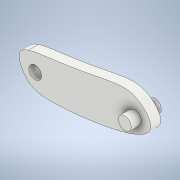
# Autodesk Inventor part: Component19
Saved by Autodesk Inventor 2022 (Build 260153000, 153)
## iProperties
Created: 2022-01-29
Part Number: Component19
Material: Generic
Document SubType Name: Modeling
Designer: Administrator
Density: 1 g/cm^3
Appearance: Default
Title: Component19
Author: Administrator
Autodesk Inventor part; units mm, degrees
ref_plane "YZ Plane" through (0, 0, 0) normal (1, 0, 0) x (0, 1, 0)
ref_plane "XZ Plane" through (0, 0, 0) normal (0, 1, 0) x (-1, 0, 0)
ref_plane "XY Plane" through (0, 0, 0) normal (0, 0, 1) x (1, 0, 0)
sketch "Sketch2" plane through (0, 0, 0) normal (0, 0, 1) x (1, 0, 0)
  circle A0 centre (27.317, 4.6906) radius 3.175
  circle A1 centre (-22.2739, -0.7171) radius 3.175
  spline S0 degree 5 poles (-25.696, 7.1239) (-24.3135, 7.5683) (-21.082, 8.2832) (-15.0705, 8.982) (-6.3104, 10.138) (4.3528, 11.9769) (13.4363, 13.9305) (20.5925, 15.117) (25.9394, 14.7964) (30.0386, 12.5835) (33.9052, 9.1125) (36.1172, 5.0315) (34.7057, 0.9553) (28.5306, -2.6686) (18.3735, -5.6185) (6.0441, -7.7995) (-6.2154, -9.141) (-16.2901, -9.5548) (-23.0885, -8.7388) (-26.5534, -6.3495) (-30.0359, -1.2094) (-31.1892, 3.3544) (-29.3768, 5.617) (-27.0784, 6.6795) (-25.696, 7.1239) knots 0 0 0 0 0 0 0.05 0.1 0.15 0.2 0.25 0.3 0.35 0.4 0.45 0.5 0.55 0.6 0.65 0.7 0.75 0.8 0.85 0.9 0.95 1 1 1 1 1 1 weights 1 1 1 1 1 1 1 1 1 1 1 1 1 1 1 1 1 1 1 1 1 1 1 1 1
  point P0 (0, 0)
  constraints: 2 centre point, 1 other
extrude "Extrusion1" add sketch "Sketch2" along normal blind 5 contours A0 | S0
extrude "Extrusion2" add sketch "Sketch2" against normal blind 5 contours A0
sketch "Sketch3" plane through (0, 0, 5) normal (0, 0, 1) x (1, 0, 0)
  circle A0 centre (27.317, 4.6906) radius 3.175 projected
  circle A1 centre (-22.2739, -0.7171) radius 3.175 projected
  point P0 (0, 0)
  constraints: 1 other
extrude "Extrusion3" add sketch "Sketch3" along normal blind 5 contours A0
body "Solid1"
